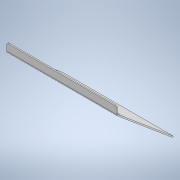
# Autodesk Inventor part: top_cover
Saved by Autodesk Inventor 2022 (Build 260153000, 153)
## iProperties
Created: 2022-08-18
Part Number: top_cover
Material: Generic
Document SubType Name: Sheet Metal
Designer: HiPeng
Density: 1 g/cm^3
Sheet Metal Rule: Default
Appearance: Default
Flat Pattern Width: 22.105 cm
Flat Pattern Length: 29.9214 cm
Flat Pattern Area: 661.412 cm^2
Sheet Metal Width: 8.703 in
Sheet Metal Length: 11.780 in
Sheet Metal Area: 102.519 in^2
Author: HiPeng
Autodesk Inventor part; units mm, degrees
ref_plane "YZ Plane" through (0, 0, 0) normal (1, 0, 0) x (0, 1, 0)
ref_plane "XZ Plane" through (0, 0, 0) normal (0, 1, 0) x (-1, 0, 0)
ref_plane "XY Plane" through (0, 0, 0) normal (0, 0, 1) x (1, 0, 0)
sketch "Sketch2" plane through (0, 0, 0) normal (0, 0, 1) x (1, 0, 0)
  line L0 (21.8354, -21.0496) -> (21.8354, -3)
  arc A0 (24.8354, 0) -> (21.8354, -3) centre (24.8354, -3) ccw
  line L1 (24.8354, 0) -> (171.4425, 0)
  line L2 (318.0496, 0) -> (171.4425, 0)
  arc A1 (321.0496, -3) -> (318.0496, 0) centre (318.0496, -3) ccw
  line L3 (321.0496, -21.0496) -> (321.0496, -3)
  line L4 (321.0496, -21.0496) -> (321.0496, -221.0496)
  line L5 (21.8354, -21.0496) -> (21.8354, -221.0496)
  line L6 (21.8354, -221.0496) -> (321.0496, -221.0496)
  point P0 (0, 0)
  dimension "d2" = 200
  dimension "d3" = 200
  measures "d2" distance of L3.start L4.end
  measures "d3" distance of L0.start L5.end
extrude "Plate1" add sketch "Sketch2" against normal blind 3.048
sketch "Sketch3" plane through (0, 0, 0) normal (0, 0, 1) x (1, 0, 0)
  line L0 (21.8354, -221.0496) -> (21.8354, -3) projected
  line L1 (321.0496, -221.0496) -> (21.8354, -221.0496) projected
  line L2 (321.0496, -3) -> (321.0496, -221.0496) projected
  arc A0 (321.0496, -3) -> (318.0496, 0) centre (318.0496, -3) ccw projected
  line L3 (24.8354, 0) -> (318.0496, 0) projected
  arc A1 (24.8354, 0) -> (21.8354, -3) centre (24.8354, -3) ccw projected
  line L4 (21.8354, -221.0496) -> (21.8354, -3) projected
  line L5 (21.8354, -21.0496) -> (321.0496, -21.0496)
  line L6 (321.0496, -3) -> (321.0496, -221.0496) projected
  point P0 (0, 0)
  dimension "d5" = 200
  constraints: 2 end point, 2 point on line, 1 perpendicular
  measures "d5" distance between parallel lines of L1 L5
fold "Fold1" angle 50 bend radius 3.048 thickness 3.048 k factor 0.44 line from (21.8354, -21.0496, 0) to (321.0496, -21.0496, 0) line at bend centre moving side (0, -1, 0) folds toward (0, 0, -1)
equation "\"d4\" = Thickness"
equation "\"d6\" = BendReliefWidth"
equation "\"d7\" = BendReliefDepth"
equation "\"d8\" = MinimumRemnant"
equation "\"d9\" = TransitionRadius"
equation "\"d11\" = BendRadius"
equation "\"BendRadius\" = Thickness"
equation "\"BendReliefWidth\" = Thickness"
equation "\"BendReliefDepth\" = 0.5 * Thickness"
equation "\"CornerReliefSize\" = 4 * Thickness"
equation "\"MinimumRemnant\" = 2 * Thickness"
equation "\"TransitionRadius\" = BendRadius"
equation "\"JacobiRadiusSize\" = BendRadius"
equation "\"GapSize\" = Thickness"
equation "\"Thickness\" = 3.048"
body "Solid2"
